Autodesk Fusion 360 part; units mm, degrees
(part 2 of 2)
sketch "Skizze21" plane through (0, 0, 0) normal (-1, 0, 0) x (0, -1, 0)
  line L0 (-20, 0) -> (0, 0)
  line L1 (0, 0) -> (0, 30)
  line L2 (0, 30) -> (-20, 30)
  line L3 (-20, 30) -> (-20, 0)
  line L4 (-20, 0) -> (-17, 0)
  line L5 (-17, 0) -> (-17, 30)
  line L6 (-17, 30) -> (-20, 30)
  line L7 (-20, 30) -> (-20, 0)
  line L8 (-20, 15) -> (0, 15) construction
  circle A0 centre (-10.5, 15) radius 1.75
  line L9 (-20, 7.5) -> (0, 7.5)
  line L10 (0, 22.5) -> (-20, 22.5)
  line L11 (-5, 0) -> (-5, 30)
  dimension "d272" = 3.5
  dimension "d273" = 9.5
  dimension "d274" = -7.5
  dimension "d275" = -7.5
  dimension "d276" = -5
  constraint horizontal L4
  constraint vertical L5
  constraint horizontal L6
  constraint vertical L7
  constraint coincident L2 L5.end
  constraint coincident L0.start L3.end
  constraint midpoint L7 L8.start
  constraint midpoint L1 L8.end
  constraint coincident L8 A0.centre
  measures "d272" diameter of A0
  measures "d273" distance of L7 A0.centre
extrude "Extrusion40" cut sketch "Skizze21" against normal blind 20 contours L0 L3 L4 L5 L7 L9 | L3 L5 L7 L9 L10 | L5 L9 L10 L11 | L2 L3 L5 L6 L7 L10 | A0 bodies 10
extrude "Extrusion41" add sketch "Skizze21" against normal blind 3.823 contours L5 L9 L10 L11 bodies 10
delete_body "Körper entfernen1" bodies 3
delete_body "Körper entfernen2" bodies 2
delete_body "Körper entfernen3" bodies 4
delete_body "Körper entfernen4" bodies 5
delete_body "Körper entfernen5" bodies 6
delete_body "Körper entfernen6" bodies 10
delete_body "Körper entfernen7" bodies 8
hidden bodies 1 7 9
equation "d6 = 14.5 mm + 5 mm"
equation "d8 = ( 5.6 / 2 ) * 1 mm"
equation "d33 = ( 5.6 / 2 ) * 1 mm"
equation "d34 = ( 5.6 / 2 ) * 1 mm"
equation "d35 = ( 5.6 / 2 ) * 1 mm"
equation "d36 = ( 5.6 / 2 ) * 1 mm"
equation "d37 = ( 5.6 / 2 ) * 1 mm"
equation "d97 = -25.8 mm + 3.05 mm"
equation "d120 = -5.5 mm - 2.5 mm"
equation "d121 = -47.7 mm - 2.5 mm"
equation "d123 = -168 mm + 50.2 mm"
equation "d133 = -168 mm + 50.2 mm"
equation "d198 = 26 mm - 14 mm"
equation "d223 = d222"
equation "d224 = 49 mm - 1.6 mm"
equation "d243 = 49 mm - 1.35 mm"
equation "d247 = -3.4 mm - 1.5 mm"
equation "d249 = -21.3 mm - 1.5 mm"
named bodies: "LargeMagnetHolder", "Unterseite Stencilhalter", "Oberseite Stencilhalter", "Handle Stencilhalter", "Stütze Stencilhalter", "Abstandhalter Stencilhalter", "PCBHolder_1.6mm", "Winkelhalter", "SmallMagnetHolder", "Oberseite Offenhalter"
